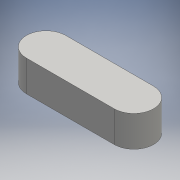
# Autodesk Inventor part: Chaveta 25
Saved by Autodesk Inventor 2016 (Build 200138000, 138)
## iProperties
Created: 2017-09-05
Part Number: Chaveta 25
Material: Genérico
Document SubType Name: Modeling
Designer: Alumno
Density: 1 g/cm^3
Appearance: Valor por defecto
Author: Alumno
Autodesk Inventor part; units mm, degrees
ref_plane "YZ Plane" through (0, 0, 0) normal (1, 0, 0) x (0, 1, 0)
ref_plane "XZ Plane" through (0, 0, 0) normal (0, 1, 0) x (-1, 0, 0)
ref_plane "XY Plane" through (0, 0, 0) normal (0, 0, 1) x (1, 0, 0)
sketch "Boceto1" plane through (0, 0, 0) normal (0, 0, 1) x (1, 0, 0)
  line L0 (8.5, -4) -> (-8.5, -4)
  line L1 (-12.5, -4) -> (-12.5, 4)
  line L2 (-8.5, 4) -> (8.5, 4)
  line L3 (12.5, 4) -> (12.5, -4)
  line L4 (-12.5, 0) -> (-8.5, 0)
  arc A0 (-8.5, 4) -> (-8.5, -4) centre (-8.5, 0) ccw
  line L5 (12.5, 0) -> (8.5, 0)
  arc A1 (8.5, -4) -> (8.5, 4) centre (8.5, 0) ccw
  point P0 (0, 0)
  dimension "d6" = 25
  dimension "d7" = 8
  dimension "d8" = 4
  dimension "d9" = 4
  constraints: 12 end point, 4 point on circle, 3 horizontal, 2 centre point, 2 coincident, 2 midpoint, 2 parallel, 2 tangent, 1 perpendicular
  measures "d6" distance of L1.end L3.start
  measures "d7" distance of L1.start L1.end
  measures "d8" distance of L4.start L4.end
  measures "d9" distance of L5.start L5.end
extrude "Extrusión2" add sketch "Boceto1" along normal blind 6
sketch "Boceto2" plane through (0, 0, 6) normal (0, 0, 1) x (1, 0, 0)
  line L0 (8.5, 4) -> (-8.5, 4) projected
  arc A0 (-8.5, 4) -> (-8.5, -4) centre (-8.5, 0) ccw projected
  line L1 (-8.5, -4) -> (8.5, -4) projected
  arc A1 (8.5, -4) -> (8.5, 4) centre (8.5, 0) ccw projected
  line L2 (-8.5, 3.8) -> (8.5, 3.8)
  arc A2 (8.5, -3.8) -> (8.5, 3.8) centre (8.5, 0) ccw
  line L3 (8.5, -3.8) -> (-8.5, -3.8)
  arc A3 (-8.5, 3.8) -> (-8.5, -3.8) centre (-8.5, 0) ccw
  point P0 (0, 0)
  dimension "d12" = 0.2
  constraints: 4 end point, 4 point on circle, 2 centre point, 3 other
  measures "d12" distance between parallel lines of L0 L2
extrude "Extrusión3" cut sketch "Boceto2" against normal blind 10
